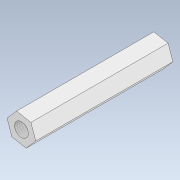
# Autodesk Inventor part: スペーサーM3L30樹脂
Saved by Autodesk Inventor 2020.2 (Build 242310000, 310)
## iProperties
Created: 2020-02-24
Part Number: スペーサーM3L30樹脂
Material: PBT プラスチック
Document SubType Name: Modeling
Designer: aoyam
Density: 1.31 g/cm^3
Appearance: 滑らか - 白
Mass: 1.08684 g
Surface Area: 7.30198 cm^2
Volume: 0.762695 cm^3
Author: aoyam
Autodesk Inventor part; units mm, degrees
ref_plane "YZ Plane" through (0, 0, 0) normal (1, 0, 0) x (0, 1, 0)
ref_plane "XZ Plane" through (0, 0, 0) normal (0, 1, 0) x (-1, 0, 0)
ref_plane "XY Plane" through (0, 0, 0) normal (0, 0, 1) x (1, 0, 0)
sketch "スケッチ1" plane through (0, 0, 0) normal (0, 0, 1) x (1, 0, 0)
  circle A0 centre (0, 0) radius 3
  circle A1 centre (0, 0) radius 1.5
  line L0 (2.0761, 2.4027) -> (3.1189, -0.5966)
  line L1 (3.1189, -0.5966) -> (1.0427, -2.9993)
  line L2 (1.0427, -2.9993) -> (-2.0761, -2.4027)
  line L3 (-2.0761, -2.4027) -> (-3.1189, 0.5966)
  line L4 (-3.1189, 0.5966) -> (-1.0427, 2.9993)
  line L5 (-1.0427, 2.9993) -> (2.0761, 2.4027)
  dimension "d0" = 6
  dimension "d1" = 3
  dimension "d13" = 5.5
  constraints: 12 end point, 3 coincident, 2 centre point, 13 other
  measures "d0" diameter of A0
  measures "d1" diameter of A1
  measures "d13" distance between parallel lines of L2 L5
extrude "押し出し1" add sketch "スケッチ1" along normal blind 30 contours L0 A0 L1 L2 L3 L4 L5 | A0 L5 L0 | L0 L1 A0 | A0 L4 L5 | L1 L2 A0 | A0 L3 L4 | L2 L3 A0
thread "ねじ1" size "M3x0.5" class "6H" standard "ANSI Metric M Profile" length 100
extrude "押し出し2" add sketch "スケッチ1" along normal blind 24 contours A1
extrude "押し出し3" cut sketch "スケッチ1" along normal blind 6 contours A1
thread "ねじ2" size "M3x0.5" class "6H" standard "ANSI Metric M Profile" full length
